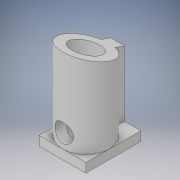
# Autodesk Inventor part: tige_ejection_douille
Saved by Autodesk Inventor 2019 (Build 230136000, 136)
## iProperties
Created: 2019-03-25
Part Number: tige_ejection_douille
Material: Générique
Document SubType Name: Modeling
Designer: theor
Density: 1 g/cm^3
Appearance: Par défaut
Author: theor
Autodesk Inventor part; units mm, degrees
ref_plane "YZ Plane" through (0, 0, 0) normal (1, 0, 0) x (0, 1, 0)
ref_plane "XZ Plane" through (0, 0, 0) normal (0, 1, 0) x (-1, 0, 0)
ref_plane "XY Plane" through (0, 0, 0) normal (0, 0, 1) x (1, 0, 0)
sketch "Esquisse1" plane through (0, 0, 0) normal (0, 1, 0) x (-1, 0, 0)
  circle A0 centre (0, 0) radius 2.5
  line L0 (0.75, -2.3848) -> (-0.75, -2.3848)
  line L1 (-0.75, -2.3848) -> (-0.75, -3.3848)
  line L2 (-0.75, -3.3848) -> (0.75, -3.3848)
  line L3 (0.75, -3.3848) -> (0.75, -2.3848)
  circle A1 centre (0, 0) radius 1.5
  dimension "d0" = 5
  dimension "d1" = 1.5
  dimension "d2" = 1
  dimension "d3" = 3
  constraints: 8 end point, 2 centre point, 2 coincident, 2 parallel, 2 point on circle, 1 horizontal, 1 perpendicular
  measures "d0" diameter of A0
  measures "d1" distance of L0.start L0.end
  measures "d2" distance of L0.end L1.end
  measures "d3" diameter of A1
extrude "Extrusion1" add sketch "Esquisse1" along normal blind 9
sketch "Esquisse2" plane through (0, 0, 0) normal (0, -1, 0) x (1, 0, 0)
  circle A0 centre (0, 0) radius 1.5 projected
  line L0 (-0.75, -3.3848) -> (-0.75, -2.3848) projected
  line L1 (0.75, -3.3848) -> (-0.75, -3.3848) projected
  line L2 (0.75, -2.3848) -> (0.75, -3.3848) projected
  arc A1 (0.75, -2.3848) -> (-0.75, -2.3848) centre (0, 0) ccw projected
  line L3 (2.5, 2.5) -> (-2.5, 2.5)
  line L4 (-2.5, 2.5) -> (-2.5, -3.3848)
  line L5 (-2.5, -3.3848) -> (2.5, -3.3848)
  line L6 (2.5, -3.3848) -> (2.5, 2.5)
  arc A2 (0.75, -2.3848) -> (-0.75, -2.3848) centre (0, 0) ccw projected
  constraints: 8 end point, 3 tangent, 2 parallel, 1 horizontal, 1 perpendicular, 1 point on line
extrude "Extrusion2" add sketch "Esquisse2" along normal blind 1
sketch "Esquisse3" plane through (0, 0, 0) normal (0, 0, 1) x (1, 0, 0)
  circle A0 centre (0, 1.5) radius 1
  line L0 (1.5, -1) -> (-1.5, -1) projected
  point P0 (0, 0)
  dimension "d8" = 2
  dimension "d9" = 2.5
  constraints: 1 centre point, 1 vertical alignment
  measures "d8" diameter of A0
  measures "d9" distance from line of A0.centre L0
extrude "Extrusion3" cut sketch "Esquisse3" along normal up to surface
sketch "Esquisse4" plane through (0, 0, 0) normal (1, 0, 0) x (0, 1, 0)
  line L0 (0, 2.5) -> (9, 2.5) projected
  line L1 (9, 2.5) -> (7, -3.3848)
  line L2 (0, -3.3848) -> (9, -3.3848) projected
  line L3 (9, 2.5) -> (9, -3.3848)
  line L4 (7, -3.3848) -> (9, -3.3848)
  point P0 (0, 0)
  dimension "d13" = 2
  constraints: 6 end point, 1 collinear, 1 point on line, 1 vertical
  measures "d13" distance of L1.end L2.end
extrude "Extrusion4" cut sketch "Esquisse4" along normal mid plane 6
